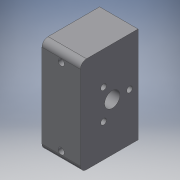
# Autodesk Inventor part: Z Leadcrew Nut Holder
Saved by Autodesk Inventor 2019 (Build 230136000, 136)
## iProperties
Created: 2020-03-07
Part Number: Z Leadcrew Nut Holder
Material: Generic
Document SubType Name: Modeling
Designer: Vijay
Density: 1 g/cm^3
Appearance: Default
Author: Vijay
Autodesk Inventor part; units mm, degrees
ref_plane "YZ Plane" through (0, 0, 0) normal (1, 0, 0) x (0, 1, 0)
ref_plane "XZ Plane" through (0, 0, 0) normal (0, 1, 0) x (-1, 0, 0)
ref_plane "XY Plane" through (0, 0, 0) normal (0, 0, 1) x (1, 0, 0)
sketch "Sketch1" plane through (0, 0, 0) normal (1, 0, 0) x (0, 1, 0)
  line L0 (176.3757, 0) -> (126.3757, 0)
  line L1 (126.3757, 0) -> (126.3757, 30)
  line L2 (126.3757, 30) -> (176.3757, 30)
  line L3 (176.3757, 30) -> (176.3757, 0)
  point P0 (0, 0)
  dimension "d0" = 30
  dimension "d1" = 50
  constraints: 8 end point, 2 parallel, 1 horizontal, 1 perpendicular
  measures "d0" distance between parallel lines of L2 L0
  measures "d1" distance of L1.end L2.end
extrude "Extrusion1" add sketch "Sketch1" along normal blind 20
fillet "Fillet1" radius 3.175 2 edges at (10, 126.3757, 30) (10, 176.3757, 30)
sketch "Sketch2" plane through (0, 129.5507, 30) normal (0, 0, 1) x (1, 0, 0)
  line L0 (0, 46.825) -> (20, 46.825) construction
  line L1 (10, 46.825) -> (10, -3.175) construction
  line L2 (0, -3.175) -> (20, -3.175) construction
  circle A0 centre (10, 41.825) radius 1.65
  circle A1 centre (10, 1.825) radius 1.65
  point P0 (0, -129.5507)
  dimension "d5" = 3.3
  dimension "d6" = 5
  dimension "d7" = 3.3
  dimension "d8" = 5
  constraints: 2 centre point, 2 end point, 2 midpoint, 2 point on line
  measures "d5" diameter of A0
  measures "d6" distance from line of L0 A0.centre
  measures "d7" diameter of A1
  measures "d8" distance from line of L2 A1.centre
extrude "Extrusion2" cut sketch "Sketch2" against normal blind 30
sketch "Sketch3" plane through (20, 0, 0) normal (1, 0, 0) x (0, 0, -1)
  line L0 (-30, 173.2007) -> (-30, 129.5507) construction
  line L1 (-30, 151.3757) -> (12.6673, 151.3757) construction
  line L2 (-26.825, 126.3757) -> (0, 126.3757) construction
  line L3 (-13.4125, 126.3757) -> (-13.4125, 176.3636) construction
  circle A0 centre (-13.4125, 151.3696) radius 4
  point P0 (0, 0)
  dimension "d11" = 8
  constraints: 4 end point, 3 midpoint, 1 centre point, 1 horizontal, 1 vertical
  measures "d11" diameter of A0
extrude "Extrusion3" cut sketch "Sketch3" against normal through all
sketch "Sketch4" plane through (20, 0, 0) normal (1, 0, 0) x (0, 0, -1)
  circle A0 centre (-13.4125, 151.3696) radius 12.5 construction
  circle A1 centre (-17.5297, 159.3727) radius 1.5 construction
  circle A2 centre (-13.4125, 151.3696) radius 5 construction
  circle A3 centre (-4.4231, 150.9337) radius 1.5 construction
  circle A4 centre (-18.2848, 143.8026) radius 1.5 construction
  circle A5 centre (-13.4125, 151.3696) radius 9 construction
  circle A6 centre (-4.4125, 151.3696) radius 1.5
  circle A7 centre (-17.9125, 159.1639) radius 1.5
  circle A8 centre (-17.9125, 143.5754) radius 1.5
  point P0 (0, 0)
  dimension "d16" = 360
  constraints: 4 centre point, 2 point on circle, 1 coincident, 1 equal radius, 7 other
extrude "Extrusion4" cut sketch "Sketch4" against normal through all
body "Solid1"
